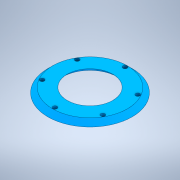
# Autodesk Inventor part: Ring_New
Saved by Autodesk Inventor 2020 (Build 240168000, 168)
## iProperties
Created: 2019-12-06
Part Number: Ring_New
Material: Generic
Document SubType Name: Modeling
Designer: Alex
Density: 1 g/cm^3
Appearance: Default(1)
Author: Alex
Autodesk Inventor part; units mm, degrees
ref_plane "YZ Plane" through (0, 0, 0) normal (1, 0, 0) x (0, 1, 0)
ref_plane "XZ Plane" through (0, 0, 0) normal (0, 1, 0) x (-1, 0, 0)
ref_plane "XY Plane" through (0, 0, 0) normal (0, 0, 1) x (1, 0, 0)
sketch "Sketch1" plane through (0, 0, 0) normal (0, 0, 1) x (1, 0, 0)
  line L0 (0, 0) -> (0, 4)
  line L1 (-23.5, 0) -> (-36, 0)
  line L2 (-36, 0) -> (-32, 4)
  line L3 (-32, 4) -> (-19.5, 4)
  line L4 (-19.5, 4) -> (-23.5, 2)
  line L5 (-23.5, 2) -> (-23.5, 0)
  point P0 (-29.75, 0)
  dimension "d0" = 47
  dimension "d1" = 12.5
  dimension "d2" = 2
  dimension "d3" = 4
  dimension "d4" = 2
  dimension "d5" = 45
  constraints: 12 end point, 2 horizontal alignment, 2 vertical, 1 horizontal, 1 midpoint, 1 parallel
  measures "d0" diameter of L5 L0
  measures "d1" distance of L1.start L1.end
  measures "d2" distance of L4.end L1.start
  measures "d3" horizontal distance of L3.end L4.end
  measures "d4" vertical distance of L3.end L4.end
  measures "d5" angle of L1 L2
revolve "Revolution1" add sketch "Sketch1" angle 360 about axis through (0, 0, 0) along (0, 1, 0)
sketch "Sketch2" plane through (0, 4, 0) normal (0, 1, 0) x (1, 0, 0)
  circle A0 centre (0, 0) radius 23.5 construction
  circle A1 centre (0, 0) radius 36 construction
  point P0 (0, -30)
  point P1 (25.9808, -15)
  point P2 (25.9808, 15)
  point P3 (0, 30)
  point P4 (-25.9808, 15)
  point P5 (-25.9808, -15)
  dimension "d10" = 360
  dimension "d19" = 30
  constraints: 1 vertical alignment, 7 other
  measures "d19" distance of point (0, 0) point (0, -30)
hole "Hole1" at (0, 4, 30) at (25.9808, 4, 15) at (25.9808, 4, -15) at (0, 4, -30) at (-25.9808, 4, -15) at (-25.9808, 4, 15) direction (0, -1, 0) diameter 3.6 end through all clearance for "Slotted Cheese Head Screw ISO 1207" size "M3" standard "ISO"
body "Solid1"
